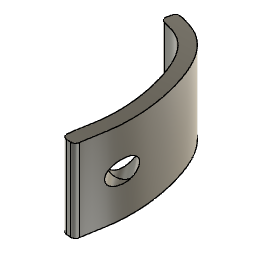
anchor point finger (Autodesk Fusion 360 design; units mm, degrees)
Autodesk Fusion 360 part; units mm, degrees
note: some values were not read from the file. Set by a fixed rule: which sketch regions a step uses.
sketch "Sketch1" plane through (0, 0, 0) normal (0, 0, 1) x (1, 0, 0)
  spline S0 degree 5 poles (4.5797, -2.6098) (4.5919, -2.5019) (4.631, -2.1851) (4.7095, -1.6645) (4.8444, -0.9397) (5.0291, 0.0374) (5.1844, 1.262) (5.2279, 2.6902) (5.1158, 4.3242) (4.8333, 6.0857) (4.3857, 7.8532) (3.7925, 9.4876) (3.0822, 10.8618) (2.2874, 11.8887) (1.4398, 12.5531) (0.6651, 12.8959) (0.0626, 13.0714) (-0.3625, 13.1791) (-0.612, 13.2403) (-0.6878, 13.2588) knots 0.032458 0.032458 0.032458 0.032458 0.032458 0.032458 0.066667 0.133333 0.2 0.266667 0.333333 0.4 0.466667 0.533333 0.6 0.666667 0.733333 0.8 0.866667 0.933333 0.96247 0.96247 0.96247 0.96247 0.96247 0.96247
  spline S1 degree 3 poles (6.0737, -2.7644) (6.167, -1.9954) (6.3349, -1.2247) (6.4898, -0.2179) (6.6681, 0.9411) (6.7693, 2.4136) (6.6093, 4.0954) (6.3711, 6.5992) (5.6092, 9.4939) (4.3777, 11.4986) (3.7289, 12.5547) (2.9028, 13.3746) (2.0449, 13.8655) (1.2137, 14.3411) (0.4372, 14.5265) (-0.2036, 14.6845) (-0.2467, 14.6952) (-0.2893, 14.7056) (-0.3316, 14.716) knots 0.033441 0.033441 0.033441 0.033441 0.196392 0.196392 0.196392 0.383976 0.383976 0.383976 0.663233 0.663233 0.663233 0.810347 0.810347 0.810347 0.95287 0.95287 0.95287 0.962447 0.962447 0.962447 0.962447
  line L0 (-0.9361, 14.3491) -> (-1.0549, 13.8633)
  line L1 (5.5396, -3.2027) -> (5.0387, -3.1648)
  arc A0 (5.5396, -3.2027) -> (6.0737, -2.7644) centre (5.5774, -2.7042) ccw
  arc A1 (4.5797, -2.6098) -> (5.0387, -3.1648) centre (5.0765, -2.6662) ccw
  arc A2 (-1.0549, 13.8633) -> (-0.6878, 13.2588) centre (-0.5692, 13.7446) ccw
  arc A3 (-0.3316, 14.716) -> (-0.9361, 14.3491) centre (-0.4504, 14.2303) ccw
  point P0 (5.1938, 2.3815)
  point P1 (2.3404, 11.729)
  dimension "d6" = 0.5
  constraint tangent S1 A0
  constraint tangent L1 A0
  constraint tangent S0 A1
  constraint tangent L1 A1
  constraint equal A0 A1
  constraint tangent L0 A2
  constraint tangent S0 A2
  constraint equal A0 A2
  constraint tangent S1 A3
  constraint tangent L0 A3
  constraint equal A0 A3
  measures "d6" radius of A0
extrude "Extrude1" add sketch "Sketch1" along normal blind 9
ref_plane "WorkPlane1" through (-0.9361, 14.349, 9) normal (-0.237549, -0.971376, 0) x (0.971376, -0.237549, 0)
sketch "Sketch2" plane through (-0.9361, 14.349, 9) normal (-0.237549, -0.971376, 0) x (0.971376, -0.237549, 0)
  circle A0 centre (2.4438, -4.7601) radius 1
  dimension "d8" = 2
  measures "d8" diameter of A0
extrude "Extrude2" cut sketch "Sketch2" along normal mid plane 3.6
ref_plane "WorkPlane2" through (0, 0, 12.125) normal (-0.573576, 0.819152, 0) x (0, 0, 1)
sketch "Sketch3" plane through (0, 0, 12.125) normal (-0.573576, 0.819152, 0) x (0, 0, 1)
  circle A0 centre (-7.625, 6.1) radius 1.2
  line L0 (-3.125, 3.3898) -> (-3.125, 10.1963)
  line L1 (-8.634, 5.4505) -> (-6.616, 5.4505)
  dimension "d12" = 2.4
  dimension "d13" = 4.5
  constraint coincident A0 L1.start
  constraint coincident A0 L1.end
  constraint perpendicular L0 L1
  measures "d12" diameter of A0
  measures "d13" distance of A0.centre L0
ref_plane "WorkPlane3" through (1.1472, -1.6383, 12.125) normal (-0.573576, 0.819152, 0) x (0, 0, 1)
sketch "Sketch4" plane through (1.1472, -1.6383, 12.125) normal (-0.573576, 0.819152, 0) x (0, 0, 1)
  circle A0 centre (-7.625, 6.1328) radius 1.25
  line L0 (-3.125, 3.3898) -> (-3.125, 10.1963)
  dimension "d15" = 2.5
  dimension "d16" = 4.5
  measures "d15" diameter of A0
  measures "d16" distance of A0.centre L0
extrude "Extrude3" cut sketch "Sketch4" along normal mid plane 10 draft -5
